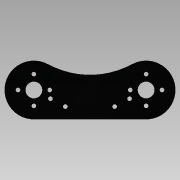
# Autodesk Inventor part: Femur3
Saved by Autodesk Inventor 2015 SP1 (Build 190203100, 203)
## iProperties
Created: 2015-01-13
Part Number: Femur3
Material: Generic
Document SubType Name: Modeling
Designer: I Was ME
Density: 1 g/cm^3
Appearance: Anodized - Black
Mass: 6.09817 g
Surface Area: 48.2309 cm^2
Volume: 6.09817 cm^3
Author: I Was ME
Autodesk Inventor part; units mm, degrees
ref_plane "YZ Plane" through (0, 0, 0) normal (1, 0, 0) x (0, 1, 0)
ref_plane "XZ Plane" through (0, 0, 0) normal (0, 1, 0) x (-1, 0, 0)
ref_plane "XY Plane" through (0, 0, 0) normal (0, 0, 1) x (1, 0, 0)
sketch "Sketch1" plane through (0, 0, 0) normal (1, 0, 0) x (0, 1, 0)
  line L0 (0, 24.9603) -> (29.0254, 24.9603)
  arc A0 (24.1037, 1.489) -> (29.0254, 24.9603) centre (30.0204, 12.5) ccw
  arc A1 (24.1037, 1.489) -> (19.8774, 3.4798) centre (-9.7194, -64.8326) ccw
  circle A2 centre (30.0204, 3.991) radius 1.25
  circle A3 centre (21.5114, 12.5) radius 1.25
  circle A4 centre (30.0204, 21.009) radius 1.25
  circle A5 centre (38.5294, 12.5) radius 1.25
  circle A6 centre (21.175, 17.1646) radius 1.25
  circle A7 centre (13.2141, 21.3627) radius 1.25
  circle A8 centre (30.0204, 12.5) radius 4.5
  line L1 (-9.7194, 24.9554) -> (-9.7296, 24.9554)
  arc A9 (-9.7194, 9.6157) -> (-9.7296, 9.6157) centre (-9.7194, -64.8326) ccw
  line L2 (-5.2398, 24.9554) -> (-5.2296, 24.9554)
  arc A10 (-5.1682, 9.6221) -> (-5.1784, 9.6221) centre (-5.1784, -64.8263) ccw
  line L3 (0, 1.489) -> (0, -13) construction
  arc A11 (-19.8774, 3.4798) -> (-24.1037, 1.489) centre (9.7194, -64.8326) ccw
  line L4 (0, 24.9603) -> (-29.0254, 24.9603)
  arc A12 (-29.0254, 24.9603) -> (-24.1037, 1.489) centre (-30.0204, 12.5) ccw
  circle A13 centre (-30.0204, 3.991) radius 1.25
  circle A14 centre (-21.5114, 12.5) radius 1.25
  circle A15 centre (-30.0204, 21.009) radius 1.25
  circle A16 centre (-38.5294, 12.5) radius 1.25
  circle A17 centre (-21.175, 17.1646) radius 1.25
  circle A18 centre (-13.2141, 21.3627) radius 1.25
  circle A19 centre (-30.0204, 12.5) radius 4.5
  line L5 (9.7194, 24.9554) -> (9.7296, 24.9554)
  arc A20 (9.7296, 9.6157) -> (9.7194, 9.6157) centre (9.7194, -64.8326) ccw
  arc A21 (5.1784, 9.6221) -> (5.1682, 9.6221) centre (5.1784, -64.8263) ccw
  line L6 (5.2398, 24.9554) -> (5.2296, 24.9554)
  arc A22 (19.8774, 3.4798) -> (-19.8774, 3.4798) centre (0, -42.3993) ccw
  arc A23 (0.2819, 5.4073) -> (-0.2819, 5.4073) centre (0, 3.4272) ccw
  arc A24 (18.5995, 0.5303) -> (-18.5995, 0.5303) centre (0, -42.3993) ccw
  arc A25 (22.6147, -1.3599) -> (18.5995, 0.5303) centre (-9.7194, -64.8326) ccw
  arc A26 (22.6147, -1.3599) -> (28.9046, 28.1747) centre (30.0204, 12.5) ccw
  line L7 (28.9046, 28.1747) -> (0, 28.1747)
  line L8 (0, 28.1747) -> (-28.9046, 28.1747)
  arc A27 (-28.9046, 28.1747) -> (-22.6147, -1.3599) centre (-30.0204, 12.5) ccw
  arc A28 (-18.5995, 0.5303) -> (-22.6147, -1.3599) centre (9.7194, -64.8326) ccw
  dimension "d47" = 8.509
  dimension "d48" = 8.509
  dimension "d49" = 8.509
  dimension "d50" = 8.509
  dimension "d51" = 10
  dimension "d53" = 9
  dimension "d56" = 9
  dimension "d58" = 4.1981
  dimension "d72" = 50
  dimension "d74" = 3.2144
  constraints: 32 point on circle, 29 centre point, 20 symmetric about line, 18 end point, 2 coincident, 2 horizontal alignment, 2 tangent, 2 vertical alignment, 1 horizontal, 1 vertical, 17 other
  measures "d47" distance of A2.centre A0.centre
  measures "d48" distance of A4.centre A0.centre
  measures "d49" distance of A5.centre A0.centre
  measures "d50" distance of A3.centre A0.centre
  measures "d51" distance of A6.centre A0.centre
  measures "d53" distance of A6.centre A7.centre
  measures "d56" diameter of A8
  measures "d58" vertical distance of A7.centre A6.centre
  measures "d72" radius of A22
  measures "d74" radial gap between concentric circles of A22 A24
extrude "Extrusion5" add sketch "Sketch1" along normal mid plane 5 contours L0 A0 A1 A22 A11 A12 L4 | A24 A28 A27 L8 L7 A26 A25
body "Solid4"
